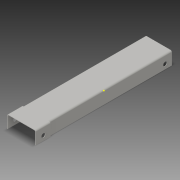
# Autodesk Inventor part: Edge
Saved by Autodesk Inventor 2016 (Build 200138000, 138)
## iProperties
Created: 2015-10-19
Part Number: Edge
Material: Generic
Document SubType Name: Sheet Metal
Designer: Rus
Density: 1 g/cm^3
Sheet Metal Rule: Default_mm
Appearance: Default
Author: Rus
Autodesk Inventor part; units mm, degrees
ref_plane "YZ Plane" through (0, 0, 0) normal (1, 0, 0) x (0, 1, 0)
ref_plane "XZ Plane" through (0, 0, 0) normal (0, 1, 0) x (-1, 0, 0)
ref_plane "XY Plane" through (0, 0, 0) normal (0, 0, 1) x (1, 0, 0)
sketch "Sketch1" plane through (0, 0, 0) normal (0, 1, 0) x (-1, 0, 0)
  line L0 (13.5, 70) -> (-13.5, 70)
  line L1 (-13.5, 70) -> (-13.5, -70)
  line L2 (-13.5, -70) -> (13.5, -70)
  line L3 (13.5, -70) -> (13.5, 70)
  line L4 (13.5, 70) -> (-13.5, -70) construction
  line L5 (-13.5, 70) -> (13.5, -70) construction
  point P0 (0, 0)
  dimension "d0" = 27
  dimension "d1" = 140
  measures "d0" distance of L0.start L0.end
  measures "d1" distance of L1.end L0.end
extrude "Plate1" add sketch "Sketch1" along normal blind 0.5
sketch "Sketch2" plane through (13, 0.5, 70) normal (1, 0, 0) x (0, 1, 0)
  line L0 (0, -140) -> (0, 0)
  line L1 (0, 0) -> (-13, 0)
  line L2 (-13, 0) -> (-13, -140)
  line L3 (-13, -140) -> (0, -140)
  constraints: 6 end point, 1 horizontal, 1 perpendicular, 1 vertical
edge flange "Flange1" height 13 angle 90 thickness 0.5 bend radius 1 thickness toward (1, 0, 0) relief straight relief width 0.5 relief depth 0.25 corner gap 0.5 corner form 0 edges at (13.5, 0, 0) (-13.5, 0, 0) wall of the first edge with corners at (13, 0.5, -70) (13, 0.5, 70) (13, -12.5, 70) (13, -12.5, -70)
bend "Bend1"
corner "Corner1"
sketch "Sketch3" plane through (13.5, -12.5, 70) normal (1, 0, 0) x (0, 0, -1)
  point P0 (70, 12.5)
sketch "Sketch4" plane through (13.5, -12.5, 70) normal (1, 0, 0) x (0, 0, -1)
  line L0 (0, 0) -> (140, 0) projected
  line L1 (0, 0) -> (7.75, 0)
  line L2 (7.75, 0) -> (7.75, 4.75)
  line L3 (7.75, 4.75) -> (0, 4.75)
  line L4 (0, 4.75) -> (0, 0)
  line L5 (0, 0) -> (132.25, 0)
  line L6 (132.25, 0) -> (132.25, 4.75)
  line L7 (132.25, 4.75) -> (0, 4.75)
  line L8 (0, 4.75) -> (0, 0)
  point P0 (70, 12.5)
  dimension "d13" = 7.75
  dimension "d14" = 4.75
  dimension "d15" = 132.25
  dimension "d16" = 4.75
  constraints: 16 end point, 4 parallel, 2 coincident, 2 horizontal, 2 perpendicular
  measures "d13" distance of L3.end L2.end
  measures "d14" distance of L2.end L1.end
  measures "d15" distance of L7.end L6.end
  measures "d16" distance of L6.end L5.end
hole "Hole1" at (13.5, -7.75, 62.25) at (13.5, -7.75, -62.25) direction (-1, 0, 0) diameter 4 end through all
sketch "Sketch5" plane through (0, 0.5, 0) normal (0, 1, 0) x (1, 0, 0)
  line L0 (-12, 70) -> (-12, -70) projected
  line L1 (12, -70) -> (-12, -70) projected
  line L2 (12, -70) -> (12, 70) projected
  line L3 (-12, 70) -> (12, 70) projected
  line L4 (-12, -70) -> (12, -70) projected
  line L5 (0, -70) -> (30, -70)
  line L6 (30, -70) -> (30, -55)
  line L7 (30, -55) -> (0, -55)
  line L8 (0, -55) -> (0, -70)
  line L9 (13.5, -60.25) -> (13.5, -64.25) projected
  line L10 (13.5, 64.25) -> (13.5, 60.25) projected
  line L11 (13.5, 70) -> (13.5, -70) projected
  line L12 (13.5, 70) -> (13.5, -70) projected
  line L13 (13.5, -60.25) -> (13.5, -64.25) projected
  line L14 (13.5, 64.25) -> (13.5, 60.25) projected
  line L15 (13.5, 70) -> (13.5, -70) projected
  line L16 (13.5, 70) -> (13.5, -70) projected
  line L17 (13.5, -60.25) -> (13.5, -64.25) projected
  line L18 (30, -55) -> (-38.1369, -55)
  line L19 (-38.1369, -55) -> (-38.1369, -70)
  line L20 (-38.1369, -70) -> (30, -70)
  line L21 (30, -70) -> (30, -55)
  point P0 (0, 0)
  dimension "d24" = 30
  dimension "d25" = 15
  constraints: 16 end point, 4 parallel, 2 horizontal, 2 perpendicular, 1 midpoint
  measures "d24" distance of L7.end L6.end
  measures "d25" distance of L5.end L6.end
extrude "Extrusion1" cut sketch "Sketch5" against normal through all contours L18 L8 L1 L0 | L0 L20 L19 L18 | L7 L2 L1 L8 | L7 L11 L9 L5 L2 | L7 L6 L5 L11 L9
sketch "Sketch6" plane through (0, 0.5, 0) normal (0, 1, 0) x (1, 0, 0)
  line L0 (0, 0) -> (0, -70)
  line L1 (0, -70) -> (0, -55)
  line L2 (12, -55) -> (-12, -55)
  line L3 (13.0625, -70) -> (13.0625, -55)
  line L4 (13.0625, -55) -> (-13.0625, -55)
  line L5 (-13.0625, -55) -> (-13.0625, -70)
  line L6 (-13.0625, -70) -> (13.0625, -70)
  line L7 (13.0625, -70) -> (-13.0625, -55) construction
  line L8 (13.0625, -55) -> (-13.0625, -70) construction
  line L9 (-12, -55) -> (-12, 70)
  line L10 (-12, -153.9917) -> (12, -153.9917)
  line L11 (12, 70) -> (12, -55)
  point P0 (0, -62.5)
  dimension "d28" = 70
  dimension "d29" = 26.125
  dimension "d53" = 24
  measures "d28" distance of L0.start L0.end
  measures "d29" distance of L4.end L3.end
  measures "d53" distance of L10.start L10.end
sheet face with bend "Face2" sketch "Sketch6" thickness 0.5 toward (0, -1, 0) bend radius 0.5 relief straight relief width 0.5 relief depth 0.25
bend "Bend2"
sketch "Sketch7" plane through (14.0625, -1, 70) normal (1, 0, 0) x (0, 1, 0)
  line L0 (0, -15) -> (0, 0)
  line L1 (0, 0) -> (-11.5, 0)
  line L2 (-11.5, 0) -> (-11.5, -15)
  line L3 (-11.5, -15) -> (0, -15)
  constraints: 6 end point, 1 horizontal, 1 perpendicular, 1 vertical
edge flange "Flange2" height 13 angle 90 thickness 0.5 bend radius 1 thickness toward (1, 0, 0) relief straight relief width 0.5 relief depth 0.25 corner gap 0.5 corner form 0 edges at (13.0625, 0, 62.5) (-13.0625, 0, 62.5) wall of the first edge with corners at (14.0625, -1, 55) (14.0625, -1, 70) (14.0625, -12.5, 70) (14.0625, -12.5, 55)
bend "Bend3"
corner "Corner2"
sketch "Sketch8" plane through (14.5625, -12.5, 70) normal (1, 0, 0) x (0, 0, -1)
  circle A0 centre (132.25, 4.75) radius 2 projected
  circle A1 centre (132.25, 4.75) radius 2 projected
  line L0 (132.25, 4.75) -> (70, 4.75)
  line L1 (70, 4.75) -> (7.75, 4.75)
  point P0 (70, 12.5)
  dimension "d45" = 62.25
  constraints: 4 end point, 1 coincident, 1 horizontal, 1 point on line
  measures "d45" distance of L0.end L1.end
hole "Hole2" at (14.5625, -7.75, 62.25) direction (-1, 0, 0) diameter 4 end through all
sketch "Sketch9" plane through (0, 0.5, 0) normal (0, 1, 0) x (1, 0, 0)
  line L0 (12, -55) -> (12, 70) projected
  line L1 (-12, 70) -> (12, 70) projected
  line L2 (-12, 70) -> (-12, -55) projected
  line L3 (-12, -55) -> (-13.0625, -55) projected
  line L4 (-13.0625, -55) -> (-13.0625, -70) projected
  line L5 (-13.0625, -70) -> (13.0625, -70) projected
  line L6 (13.0625, -70) -> (13.0625, -55) projected
  line L7 (13.0625, -55) -> (12, -55) projected
  line L8 (0, 0) -> (0, 69)
  line L9 (-38.4994, 118.6469) -> (-38.4994, 69)
  line L10 (-38.4994, 69) -> (38.4994, 69)
  line L11 (38.4994, 69) -> (38.4994, 118.6469)
  line L12 (38.4994, 118.6469) -> (-38.4994, 118.6469)
  line L13 (-38.4994, 118.6469) -> (38.4994, 69) construction
  line L14 (-38.4994, 69) -> (38.4994, 118.6469) construction
  point P0 (0, 93.8235)
  dimension "d54" = 69
  constraints: 14 end point, 3 parallel, 2 midpoint, 1 perpendicular, 1 vertical
  measures "d54" distance of L8.start L8.end
extrude "Extrusion2" cut sketch "Sketch9" against normal through all contours L10 L2 L1 L0 | L0 L1 L2 L10 L9 L12 L11
equation "\"d22\" = Thickness"
equation "\"d51\" = Thickness"
equation "\"d3\" = BendReliefWidth"
equation "\"d4\" = BendReliefDepth"
equation "\"d5\" = MinimumRemnant"
equation "\"d6\" = BendRadius"
equation "\"d10\" = CornerReliefSize"
equation "\"d11\" = GapSize"
equation "\"d12\" = JacobiRadiusSize"
equation "\"d30\" = BendRadius"
equation "\"d31\" = BendReliefWidth"
equation "\"d33\" = MinimumRemnant"
equation "\"d32\" = BendReliefDepth"
equation "\"d34\" = BendRadius"
equation "\"d35\" = BendReliefWidth"
equation "\"d36\" = BendReliefDepth"
equation "\"d37\" = MinimumRemnant"
equation "\"d38\" = BendRadius"
equation "\"d42\" = CornerReliefSize"
equation "\"d43\" = GapSize"
equation "\"d44\" = JacobiRadiusSize"
equation "\"BendRadius\" = Thickness"
equation "\"BendReliefWidth\" = Thickness"
equation "\"BendReliefDepth\" = 0.5 * Thickness"
equation "\"CornerReliefSize\" = 4 * Thickness"
equation "\"MinimumRemnant\" = 2 * Thickness"
equation "\"TransitionRadius\" = BendRadius"
equation "\"JacobiRadiusSize\" = BendRadius"
equation "\"GapSize\" = Thickness"
equation "\"d2\" = BendRadius"
equation "\"Thickness\" = 0.5"
body "Solid1"
